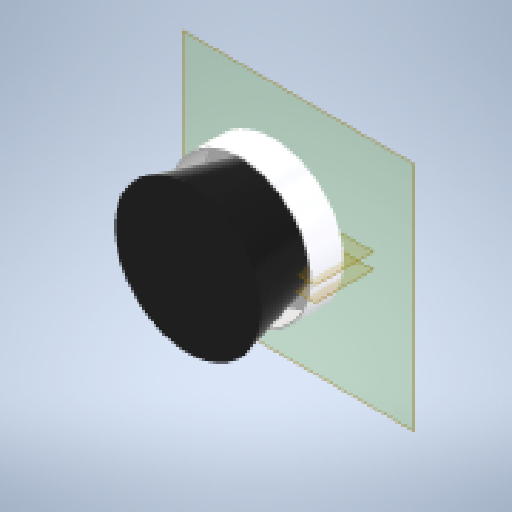
# Autodesk Inventor part: BRUSH1
Saved by Autodesk Inventor 2024 (Build 280153000, 153)
## iProperties
Created: 2024-04-11
Part Number: BRUSH1
Material: Generic
Document SubType Name: Modeling
Designer: teeta
Density: 1 g/cm^3
Appearance: Default
Author: teeta
Autodesk Inventor part; units mm, degrees
ref_plane "YZ Plane" through (0, 0, 0) normal (1, 0, 0) x (0, 1, 0)
ref_plane "XY Plane" through (0, 0, 0) normal (0, 0, 1) x (1, 0, 0)
ref_plane "Work Plane1" through (0, 0, -0.5) normal (0, 0, -1) x (-1, 0, 0)
sketch "Sketch1" plane through (0, 0, -0.5) normal (0, 0, -1) x (-1, 0, 0)
  line L0 (134.0347, 37.6976) -> (134.0347, -12.3024) projected
  line L1 (134.0347, 37.6976) -> (30.0097, 37.6976) projected
  line L2 (30.0097, 37.6976) -> (30.0097, 128.6976) projected
  line L3 (-19.9903, 128.6976) -> (30.0097, 128.6976) projected
  line L4 (-19.9903, 128.6976) -> (-19.9903, 37.6976) projected
  line L5 (-19.9903, 37.6976) -> (-140.9903, 37.6976) projected
  line L6 (-140.9903, -12.3024) -> (-140.9903, 37.6976) projected
  line L7 (-140.9903, -12.3024) -> (-19.9903, -12.3024) projected
  line L8 (-19.9903, -12.3024) -> (-19.9903, -146.3274) projected
  line L9 (30.0097, -146.3274) -> (-19.9903, -146.3274) projected
  line L10 (30.0097, -146.3274) -> (30.0097, -12.3024) projected
  line L11 (30.0097, -12.3024) -> (134.0347, -12.3024) projected
  line L12 (-19.9903, 37.6976) -> (30.0097, -12.3024) construction
  line L13 (30.0097, 37.6976) -> (-19.9903, -12.3024) construction
  circle A0 centre (5.0097, 12.6976) radius 20
  point P0 (0, 0)
  dimension "d0" = 40
  constraints: 4 end point, 1 centre point, 1 midpoint, 1 perpendicular, 1 point on line
  measures "d0" diameter of A0
extrude "Extrusion1" add sketch "Sketch1" against normal blind 25.75 contours A0
sketch "Sketch2" plane through (-5.0097, 12.6976, 25.25) normal (0, 0, 1) x (1, 0, 0)
  circle A0 centre (0, 0) radius 92.639
  point P0 (5.0097, -12.6976)
  constraints: 1 centre point
extrude "Extrusion2" add sketch "Sketch2" along normal blind 42.75
shell "Shell1" thickness 2 removed faces 1 at (-24.2409, 34.4376, 68)
ref_plane "Work Plane3" through (-5.0097, 12.6976, -0.5) normal (0, 1, 0) x (-1, 0, 0)
ref_plane "Work Plane2" through (-5.0097, -7.3024, -0.5) normal (0, 1, 0) x (-1, 0, 0)
sketch "Sketch3" plane through (-5.0097, 12.6976, -0.5) normal (0, 1, 0) x (-1, 0, 0)
  line L0 (18, 27.75) -> (-18, 27.75) projected
  line L1 (0, 27.75) -> (-68, 27.75)
  line L2 (90.639, 27.75) -> (-90.639, 27.75) projected
  line L3 (-68, 27.75) -> (-95.6652, 136.8622)
  line L4 (-95.6652, 136.8622) -> (0, 136.8622)
  line L5 (0, 136.8622) -> (0, 27.75)
  point P0 (-5.0097, 0.5)
  dimension "d8" = 95.6652
  dimension "d9" = 68
  constraints: 8 end point, 1 midpoint, 1 parallel, 1 perpendicular, 1 point on line
  measures "d8" distance of L3.end L4.end
  measures "d9" distance of L1.start L1.end
revolve "Revolution1" add sketch "Sketch3" angle 360 about axis through (-5.0097, 12.6976, 136.3622) along (0, 0, -1)
sketch "Sketch4" plane through (-5.0097, 12.6976, -0.5) normal (0, 0, -1) x (-1, 0, 0)
  circle A0 centre (0, 0) radius 20 projected
  point P0 (-5.0097, -12.6976)
extrude "Extrusion3" add sketch "Sketch4" along normal blind 24.25
body "Solid1"
